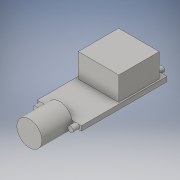
# Autodesk Inventor part: Motor Driver
Saved by Autodesk Inventor 2016 (Build 200138000, 138)
## iProperties
Created: 2018-02-08
Part Number: Motor Driver
Material: Generic
Document SubType Name: Modeling
Designer: Student
Density: 1 g/cm^3
Appearance: Default
Author: Student
Autodesk Inventor part; units mm, degrees
ref_plane "YZ Plane" through (0, 0, 0) normal (1, 0, 0) x (0, 1, 0)
ref_plane "XZ Plane" through (0, 0, 0) normal (0, 1, 0) x (-1, 0, 0)
ref_plane "XY Plane" through (0, 0, 0) normal (0, 0, 1) x (1, 0, 0)
sketch "Sketch1" plane through (0, 0, 0) normal (0, 1, 0) x (-1, 0, 0)
  line L0 (16.1537, 17.2566) -> (-1.9057, 17.2566)
  line L1 (-1.9057, 17.2566) -> (-1.9057, -17.516)
  line L2 (-1.9057, -17.516) -> (16.1537, -17.516)
  line L3 (16.1537, -17.516) -> (16.1537, 17.2566)
  point P0 (0, 0)
  dimension "d0" = 34.7726
  dimension "d1" = 18.0594
  constraints: 8 end point, 2 parallel, 1 horizontal, 1 perpendicular
  measures "d0" distance of L2.end L0.start
  measures "d1" distance of L1.end L2.end
extrude "Extrusion1" add sketch "Sketch1" along normal blind 1.9304
sketch "Sketch2" plane through (0, 1.9304, 0) normal (0, 1, 0) x (1, 0, 0)
  line L0 (-15.2139, -1.4832) -> (1.2961, -1.4832)
  line L1 (1.2961, -1.4832) -> (1.2961, 14.976)
  line L2 (1.2961, 14.976) -> (-15.2139, 14.976)
  line L3 (-15.2139, 14.976) -> (-15.2139, -1.4832)
  line L4 (1.9057, -17.2566) -> (1.9057, 17.516) projected
  line L5 (1.9057, 17.516) -> (-16.1537, 17.516) projected
  line L6 (-16.1537, -17.2566) -> (1.9057, -17.2566) projected
  point P0 (0, 0)
  dimension "d4" = 16.4592
  dimension "d5" = 16.51
  dimension "d6" = 0.6096
  dimension "d9" = 15.7734
  constraints: 8 end point, 2 parallel, 1 horizontal, 1 perpendicular
  measures "d4" distance of L2.end L0.start
  measures "d5" distance of L1.end L2.end
  measures "d6" distance between parallel lines of L1 L4
  measures "d9" distance between parallel lines of L6 L0
extrude "Extrusion2" add sketch "Sketch2" along normal blind 9.6774
sketch "Sketch3" plane through (-16.1537, 0, 17.2566) normal (0, 0, 1) x (1, 0, 0)
  line L0 (17.4498, 1.9304) -> (0.9398, 1.9304) projected
  line L1 (9.1948, 1.9304) -> (9.1948, -4.4517)
  line L2 (18.0594, 0) -> (18.0594, 1.9304) projected
  line L3 (18.0594, 0.9652) -> (-4.716, 0.9652)
  circle A0 centre (9.1948, 0.9652) radius 5.08
  point P0 (16.1537, 0)
  dimension "d12" = 10.16
  constraints: 4 end point, 2 midpoint, 2 point on line, 1 centre point, 1 horizontal, 1 vertical
  measures "d12" diameter of A0
extrude "Extrusion3" add sketch "Sketch3" along normal blind 12.3444
sketch "Sketch4" plane through (1.9057, 0, -17.516) normal (0, 0, -1) x (-1, 0, 0)
  line L0 (0, 0) -> (0, 1.9304) projected
  line L1 (0, 0.9652) -> (18.0594, 0.9652)
  line L2 (18.0594, 0) -> (18.0594, 1.9304) projected
  line L3 (13.8521, 1.9304) -> (3.8771, 1.9304) projected
  line L4 (8.8646, 1.9304) -> (8.8646, -5.2451)
  line L5 (18.0594, 1.3992) -> (13.462, 1.3992)
  line L6 (13.462, 1.9304) -> (13.462, -4.7459)
  line L7 (0, 1.6034) -> (4.5974, 1.6034)
  line L8 (4.5974, 1.9304) -> (4.5974, -5.3585)
  circle A0 centre (4.5974, 0.9652) radius 1.1176
  circle A1 centre (8.8646, 0.9652) radius 1.1176
  circle A2 centre (13.462, 0.9652) radius 1.1176
  point P0 (1.9057, 0)
  dimension "d15" = 9.1948
  dimension "d16" = 4.5974
  dimension "d17" = 4.5974
  dimension "d18" = 2.2352
  dimension "d19" = 2.2352
  dimension "d20" = 2.2352
  constraints: 12 end point, 10 point on line, 3 centre point, 3 midpoint, 2 perpendicular, 2 vertical, 1 horizontal
  measures "d15" distance between parallel lines of L2 L4
  measures "d16" distance of L5.start L5.end
  measures "d17" distance of L7.start L7.end
  measures "d18" diameter of A0
  measures "d19" diameter of A1
  measures "d20" diameter of A2
extrude "Extrusion4" add sketch "Sketch4" along normal blind 2.54 contours A0 L7 L8 L1 | L1 L8 A0 | A0 L3 L8 L7 | L8 L3 A0 L1 | L1 A0 L8 | A0 L3 | A1 L3 L4 L1 | L1 L4 A1 | A1 L3 | L4 L3 A1 L1 | L1 A1 L4 | A2 L5 L6 L3 | L3 L6 L1 A2 | L1 L6 A2 | A2 L1 L6 L5 | L1 A2 L6
sketch "Sketch5" plane through (1.9057, 0, 17.2566) normal (0, 0, 1) x (1, 0, 0)
  circle A0 centre (-1.9057, 0.9652) radius 1.1147
  circle A1 centre (-16.0424, 0.9652) radius 1.1215
  point P0 (-1.9057, 0)
  constraints: 2 centre point
extrude "Extrusion5" add sketch "Sketch5" along normal blind 2.54
equation "\"d19\" = d18"
equation "\"d20\" = d18"
body "Solid1"
